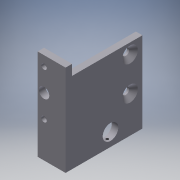
# Autodesk Inventor part: Motorhalter
Saved by Autodesk Inventor 2018 (Build 220112000, 112)
## iProperties
Created: 2013-02-20
Part Number: Motorhalter
Material: Aluminum-6061
Document SubType Name: Modeling
Designer: Neef
Mass: 45.4065 g
Surface Area: 81.6955 cm^2
Volume: 16.7552 cm^3
Density: 2.71 g/cm^3
Appearance: Aluminum - Flat
Author: Neef
Autodesk Inventor part; units mm, degrees
note: some values were not read from the file. Chosen so that the rebuilt part matches the saved one: direction of "Bohrung3".
ref_plane "YZ Plane" through (0, 0, 0) normal (1, 0, 0) x (0, 1, 0)
ref_plane "XZ Plane" through (0, 0, 0) normal (0, 1, 0) x (-1, 0, 0)
ref_plane "XY Plane" through (0, 0, 0) normal (0, 0, 1) x (1, 0, 0)
sketch "Skizze1" plane through (0, 0, 0) normal (0, 0, 1) x (1, 0, 0)
  line L0 (0, 70.8) -> (0, -11.8) projected
  line L1 (-25.8, 0) -> (4.3, 0) projected
  line L2 (-21.5, 0) -> (-21.5, 5)
  line L3 (-21.5, 5) -> (-5, 5)
  line L4 (-5, 5) -> (-5, 59)
  line L5 (-5, 59) -> (0, 59)
  line L6 (0, 59) -> (0, 0)
  line L7 (0, 0) -> (-21.5, 0)
  dimension "d0" = 16.5
  dimension "d1" = 5
  dimension "d2" = 5
  dimension "d3" = 54
  constraints: 12 end point, 4 perpendicular, 2 point on line, 1 collinear, 1 parallel
  measures "d0" distance of L2.end L3.end
  measures "d1" distance of L4.end L5.end
  measures "d2" distance of L2.start L2.end
  measures "d3" distance of L3.end L4.end
extrude "Extrusion1" add sketch "Skizze1" along normal blind 70
sketch "Skizze2" plane through (-21.5, 5, 0) normal (0, 1, 0) x (1, 0, 0)
  line L0 (0, -70) -> (16.5, -70) projected
  line L1 (0, 0) -> (0, -70) projected
  point P0 (21.5, 0)
  point P1 (5, -62.5)
  point P2 (5, -27.5)
  dimension "d6" = 35
  dimension "d7" = 5
  dimension "d8" = 5
  dimension "d9" = 7.5
  measures "d6" distance of point (5, -62.5) point (5, -27.5)
  measures "d7" distance from line of point (5, -62.5) L1
  measures "d8" distance from line of point (5, -27.5) L1
  measures "d9" distance from line of L0 point (5, -62.5)
hole "Bohrung1" at (-16.5, 5, 62.5) at (-16.5, 5, 27.5) direction (0, -1, 0) diameter 4.2 end through all countersink diameter 9 countersink angle 90 clearance for "Innensechskant-Senkkopfschraube DIN EN ISO 10642" size "M4" standard "DIN"
sketch "Skizze3" plane through (-21.5, 5, 0) normal (0, 1, 0) x (1, 0, 0)
  circle A0 centre (5, -27.5) radius 4.5 projected
  circle A1 centre (5, -62.5) radius 4.5 projected
  line L0 (0, 0) -> (0, -70) projected
  line L1 (5, -62.5) -> (5, -27.5) construction
  circle A2 centre (5, -45) radius 4
  point P0 (21.5, 0)
  dimension "d18" = 17.5
  dimension "d19" = 8
  constraints: 2 end point, 1 centre point, 1 coincident, 1 midpoint, 1 parallel
  measures "d18" distance of point (5, -45) L1.start
  measures "d19" diameter of A2
extrude "Extrusion2" cut sketch "Skizze3" against normal up to surface (5 mm away) contours A2
sketch "Skizze4" plane through (0, 0, 0) normal (1, 0, 0) x (0, 0, -1)
  line L0 (-70, 59) -> (-70, 0) projected
  line L1 (0, 59) -> (-70, 59) projected
  circle A0 centre (-34, 39.5) radius 2.067 projected
  circle A1 centre (-8, 39.5) radius 2.067 projected
  point P0 (-54, 49.5)
  point P1 (-28, 49.5)
  dimension "d34" = 9.5
  dimension "d35" = 9.5
  dimension "d36" = 16
  dimension "d37" = 26
  measures "d34" distance from line of L1 point (-54, 49.5)
  measures "d35" distance from line of L1 point (-28, 49.5)
  measures "d36" distance from line of L0 point (-54, 49.5)
  measures "d37" distance of point (-28, 49.5) point (-54, 49.5)
hole "Bohrung2" at (0, 49.5, 54) at (0, 49.5, 28) direction (-1, 0, 0) diameter 5.3 end through all countersink diameter 12 countersink angle 90 clearance for "Innensechskant-Senkkopfschraube DIN EN ISO 10642" size "M5" standard "DIN"
sketch "Skizze5" plane through (-5, 5, 0) normal (-1, 0, 0) x (0, 0, 1)
  line L0 (0, 54) -> (70, 54) projected
  line L1 (0, 54) -> (0, 0) projected
  circle A0 centre (10, 29.5) radius 6
  circle A1 centre (28, 44.5) radius 2.067 projected
  circle A2 centre (54, 44.5) radius 2.067 projected
  circle A3 centre (18.5, 60.5) radius 2.2 projected
  line L2 (62, 72) -> (62, 35) projected
  line L3 (62, 72) -> (-5.5, 72) projected
  arc A4 (-28, 90.2303) -> (-5.5, 72) centre (-5.5, 95) ccw projected
  line L4 (-28, 15) -> (-28, 90.2303) projected
  line L5 (-28, 15) -> (-18, 15) projected
  line L6 (-18, 35) -> (-18, 15) projected
  line L7 (62, 35) -> (-18, 35) projected
  circle A5 centre (28, 44.5) radius 2.65 projected
  circle A6 centre (54, 44.5) radius 2.65 projected
  line L8 (70, 0) -> (70, 54) projected
  line L9 (0, 54) -> (70, 54) projected
  line L10 (0, 54) -> (0, 0) projected
  line L11 (0, 0) -> (70, 0) projected
  line L12 (32.75, 18) -> (32.75, 106)
  point P0 (0, -5)
  dimension "d38" = 24.5
  dimension "d39" = 12
  dimension "d40" = 10
  constraints: 2 end point, 1 centre point, 1 vertical, 2 other
  measures "d38" distance from line of L0 A0.centre
  measures "d39" diameter of A0
  measures "d40" distance from line of A0.centre L1
extrude "Extrusion3" cut sketch "Skizze5" against normal blind 5 contours L7 A0 | A0 L7
sketch "Skizze7" plane through (0, 0, 0) normal (0, 0, -1) x (-1, 0, 0)
  line L0 (0, 28.5) -> (0, 40.5) projected
  line L1 (0, 28.5) -> (0, 40.5) projected
  line L2 (5, 40.5) -> (5, 28.5) projected
  line L3 (5, 28.5) -> (0, 28.5) projected
  line L4 (5, 40.5) -> (0, 40.5) projected
  point P0 (2.5, 34.5)
hole "Bohrung3" at (-2.5, 34.5, 0) direction (0, 0, 1) diameter 2.013 end up to surface thread size "M2.5x0.45" class "6H" standard "ISO Metric profile"
sketch "Skizze8" plane through (-5, 5, 0) normal (-1, 0, 0) x (0, 0, 1)
  line L0 (0, 0) -> (70, 0) projected
  line L1 (70, 54) -> (62, 54)
  line L2 (62, 54) -> (62, 0)
  line L3 (62, 0) -> (70, 0)
  line L4 (70, 0) -> (70, 54)
  point P0 (0, -5)
  dimension "d50" = 8
  constraints: 8 end point, 2 parallel, 1 horizontal, 1 perpendicular, 1 point on line
  measures "d50" distance between parallel lines of L4 L2
extrude "Extrusion4" cut sketch "Skizze8" against normal blind 5
equation "\"d2\" = d1"
equation "\"d8\" = d7"
equation "\"d35\" = d34"
